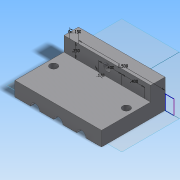
# Autodesk Inventor part: keyhole holder-01
Saved by Autodesk Inventor 2014 SP2 (Build 180246200, 246)
## iProperties
Created: 2014-06-06
Part Number: keyhole holder-01
Material: Generic
Document SubType Name: Modeling
Designer: dliu
Density: 1 g/cm^3
Appearance: Default
Author: dliu
Autodesk Inventor part; units mm, degrees
ref_plane "YZ Plane" through (0, 0, 0) normal (1, 0, 0) x (0, 1, 0)
ref_plane "XZ Plane" through (0, 0, 0) normal (0, 1, 0) x (-1, 0, 0)
ref_plane "XY Plane" through (0, 0, 0) normal (0, 0, 1) x (1, 0, 0)
sketch "Sketch1" plane through (0, 0, 0) normal (0, 0, 1) x (1, 0, 0)
  circle A0 centre (-10.16, 0) radius 2.2543
  circle A1 centre (0, 0) radius 2.2543
  circle A2 centre (10.16, 0) radius 2.2543
  line L0 (-19.05, 6.35) -> (19.05, 6.35)
  line L1 (19.05, 6.35) -> (19.05, 0)
  line L2 (19.05, 0) -> (-19.05, 0)
  line L3 (-19.05, 0) -> (-19.05, 6.35)
  dimension "d0" = 4.5085
  dimension "d3" = 10.16
  dimension "d4" = 10.16
  dimension "d5" = 6.35
  dimension "d6" = 38.1
  constraints: 8 end point, 3 centre point, 3 horizontal alignment, 2 equal radius, 2 parallel, 1 coincident, 1 horizontal, 1 midpoint, 1 perpendicular
  measures "d0" diameter of A0
  measures "d3" distance of A1.centre A0.centre
  measures "d4" distance of A2.centre A1.centre
  measures "d5" distance of L2.end L0.start
  measures "d6" distance of L0.start L0.end
extrude "Extrusion1" add sketch "Sketch1" along normal blind 27.94 contours L2 A0 | A0 L2 L3 L0 L1 A2 A1 | A1 L2 | A2 L2 picked at (-10.9114, 0.6984) picked at (0.5625, 0.4983) picked at (9.4728, 0.529)
extrude "Extrusion2" cut sketch "Sketch1" along normal blind 20.574 contours L2 A0 | A0 L2 | L2 A1 | A1 L2 | L2 A2 | A2 L2
sketch "Sketch2" plane through (0, 0, 27.94) normal (0, 0, 1) x (1, 0, 0)
  circle A0 centre (0, 0) radius 2.2543 projected
  circle A1 centre (10.16, 0) radius 2.2543 projected
  circle A2 centre (-10.16, 0) radius 2.2543 projected
  circle A3 centre (-10.16, 0) radius 2.032
  circle A4 centre (0, 0) radius 2.032
  circle A5 centre (10.16, 0) radius 2.032
  dimension "d11" = 4.064
  constraints: 3 centre point, 3 coincident, 2 equal radius
  measures "d11" diameter of A3
extrude "Extrusion3" cut sketch "Sketch2" against normal through all contours A3 | A4 | A5
sketch "Sketch3" plane through (0, 0, 0) normal (0, 1, 0) x (-1, 0, 0)
  point P0 (-16.002, 13.97)
  point P1 (0, 0)
  dimension "d38" = 13.97
  dimension "d39" = 16.002
  measures "d38" vertical distance of point (0, 0) point (-16.002, 13.97)
  measures "d39" horizontal distance of point (0, 0) point (-16.002, 13.97)
hole "Hole1" at (16.002, 0, 13.97) direction (0, 1, 0) diameter 3.2766 end through all clearance for "Oval Head Machine Screw" size "#4" standard "Ansi Unified Screw Threads"
mirror "Mirror1" about plane through (0, 0, 0) normal (1, 0, 0) of "Hole1"
sketch "Sketch7" plane through (0, 0, 0) normal (0, 0, 1) x (1, 0, 0)
  line L0 (-19.05, 6.35) -> (19.05, 6.35) projected
  line L1 (19.05, 6.35) -> (-19.05, 6.35)
  line L2 (-19.05, 6.35) -> (-19.05, 12.7)
  line L3 (-19.05, 12.7) -> (19.05, 12.7)
  line L4 (19.05, 12.7) -> (19.05, 6.35)
  point P0 (0, 10.033)
  point P1 (0, 0)
  point P2 (0, 10.033)
  dimension "d40" = 6.35
  dimension "d41" = 3.683
  constraints: 8 end point, 2 parallel, 1 coincident, 1 horizontal, 1 perpendicular, 1 vertical alignment
  measures "d40" distance between parallel lines of L0 L3
  measures "d41" distance from line of L0 point (0, 10.033)
extrude "Extrusion5" add sketch "Sketch7" along normal blind 6.35
hole "Hole2" at (0, 10.033, 0) direction (0, 0, 1) diameter 3.2766 end through all clearance for "Oval Head Machine Screw" size "#4" standard "Ansi Unified Screw Threads"
sketch "Sketch8" plane through (0, 0, 0) normal (0, 0, -1) x (-1, 0, 0)
  line L0 (19.05, 12.7) -> (19.05, 0) projected
  line L1 (-19.05, 12.7) -> (-19.05, 0) projected
  line L2 (-19.05, 12.7) -> (19.05, 12.7) projected
  line L3 (15.24, 0) -> (15.24, 16.51)
  line L4 (15.24, 16.51) -> (-22.86, 16.51)
  line L5 (-22.86, 16.51) -> (-22.86, 0)
  line L6 (-22.86, 0) -> (-19.05, 0)
  line L7 (19.05, 0) -> (15.24, 0)
  point P0 (19.05, 6.35)
  point P1 (-19.05, 6.35)
  dimension "d49" = 3.81
  constraints: 10 end point, 1 collinear, 1 perpendicular, 2 other
  measures "d49" distance between parallel lines of L2 L4
extrude "Extrusion6" [suppressed]
sketch "Sketch9" plane through (0, 0, 0) normal (0, 0, -1) x (-1, 0, 0)
  line L0 (19.05, 0) -> (19.05, 6.35) projected
  line L1 (-19.05, 6.35) -> (-19.05, 0) projected
  line L2 (-22.86, 0) -> (-22.86, 6.35)
  line L3 (22.86, 6.35) -> (22.86, 0)
  line L4 (-22.86, 0) -> (-19.05, 0)
  line L5 (19.05, 0) -> (22.86, 0)
  line L6 (-22.86, 6.35) -> (-19.05, 6.35)
  line L7 (19.05, 6.35) -> (22.86, 6.35)
  line L8 (-19.05, 6.35) -> (-19.05, 0)
  dimension "d48" = 3.81
  constraints: 14 end point, 2 equal length, 2 perpendicular, 1 horizontal
  measures "d48" distance between parallel lines of L0 L3
extrude "Extrusion7" [suppressed]
equation "\"d49\" = FlangeWidth"
equation "\"d48\" = FlangeWidth"
equation "\"FlangeWidth\" = 3.81"
body "Solid1"
